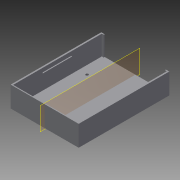
# Autodesk Inventor part: bottom1
Saved by Autodesk Inventor 2015 SP2 (Build 190223200, 223)
## iProperties
Created: 2016-03-10
Part Number: bottom1
Material: Generic
Document SubType Name: Modeling
Designer: mca20
Density: 1 g/cm^3
Appearance: Default
Author: mca20
Autodesk Inventor part; units mm, degrees
ref_plane "YZ Plane" through (0, 0, 0) normal (1, 0, 0) x (0, 1, 0)
ref_plane "XZ Plane" through (0, 0, 0) normal (0, 1, 0) x (-1, 0, 0)
ref_plane "XY Plane" through (0, 0, 0) normal (0, 0, 1) x (1, 0, 0)
sketch "Sketch1" plane through (0, 0, 0) normal (0, 1, 0) x (-1, 0, 0)
  line L0 (0, 0) -> (56, 0)
  line L1 (56, 0) -> (56, -85)
  line L2 (56, -85) -> (0, -85)
  line L3 (0, -85) -> (0, 0)
  line L4 (61, -90) -> (61, 5)
  line L5 (61, 5) -> (-5, 5)
  line L6 (-5, 5) -> (-5, -90)
  line L7 (61, -85) -> (-5, -85)
  dimension "d0" = 56
  dimension "d1" = 85
  dimension "d2" = 5
  dimension "d50" = 90
  constraints: 16 end point, 3 parallel, 3 point on line, 2 perpendicular, 1 horizontal, 2 other
  measures "d0" distance of L1.end L2.end
  measures "d1" distance of L0.end L1.end
  measures "d2" distance between parallel lines of L1 L4
  measures "d50" distance between parallel lines of L5 L2
extrude "Extrusion1" add sketch "Sketch1" along normal blind 1
sketch "Sketch2" plane through (0, 1, 0) normal (0, 1, 0) x (1, 0, 0)
  line L0 (-61, -5) -> (5, -5) projected
  line L1 (-61, 85) -> (-61, -5) projected
  line L2 (-61, -5) -> (5, -5) projected
  line L3 (5, -5) -> (5, 85) projected
  line L4 (5, 85) -> (-61, 85) projected
  line L5 (-62, 86) -> (6, 86)
  line L6 (6, 86) -> (6, -6)
  line L7 (6, -6) -> (-62, -6)
  line L8 (-62, -6) -> (-62, 86)
  point P0 (0, 0)
  dimension "d41" = 1
  constraints: 8 end point, 3 other
  measures "d41" distance between parallel lines of L4 L5
sketch "Sketch4" plane through (0, 1, 0) normal (0, 1, 0) x (1, 0, 0)
  line L0 (0, 0) -> (-56, 0)
  line L1 (-56, 0) -> (-56, 85)
  line L2 (-56, 85) -> (0, 85)
  line L3 (0, 85) -> (0, 0)
  circle A0 centre (-3.5, 3.5) radius 1.375
  circle A1 centre (-52.5, 3.5) radius 1.375
  circle A2 centre (-52.5, 61.5) radius 1.375
  circle A3 centre (-3.5, 61.5) radius 1.375
  circle A4 centre (-52.5, 3.5) radius 3.1
  circle A5 centre (-52.5, 61.5) radius 3.1
  circle A6 centre (-3.5, 3.5) radius 3.1
  circle A7 centre (-3.5, 61.5) radius 3.1
  dimension "d14" = 56
  dimension "d15" = 85
  dimension "d16" = 2.75
  dimension "d17" = 2.75
  dimension "d18" = 2.75
  dimension "d19" = 2.75
  dimension "d20" = 49
  dimension "d21" = 58
  dimension "d22" = 58
  dimension "d23" = 49
  dimension "d24" = 6.2
  dimension "d25" = 6.2
  dimension "d26" = 6.2
  dimension "d27" = 6.2
  dimension "d28" = 3.5
  dimension "d29" = 3.5
  dimension "d30" = 3.5
  dimension "d31" = 3.5
  dimension "d32" = 3.5
  constraints: 8 centre point, 8 end point, 4 coincident, 2 parallel, 1 horizontal, 1 perpendicular
  measures "d14" distance of L1.end L2.end
  measures "d15" distance of L0.end L1.end
  measures "d16" diameter of A0
  measures "d17" diameter of A1
  measures "d18" diameter of A2
  measures "d19" diameter of A3
  measures "d20" distance of A0.centre A1.centre
  measures "d21" distance of A2.centre A1.centre
  measures "d22" distance of A3.centre A0.centre
  measures "d23" distance of A3.centre A2.centre
  measures "d24" diameter of A4
  measures "d25" diameter of A5
  measures "d26" diameter of A6
  measures "d27" diameter of A7
  measures "d28" distance from line of A4.centre L1
  measures "d29" distance from line of L0 A0.centre
  measures "d30" distance from line of A2.centre L1
  measures "d31" distance from line of L3 A3.centre
  measures "d32" distance from line of L0 A1.centre
hole "Hole1" at (-52.5, 1, -61.5) at (-52.5, 1, -3.5) at (-3.5, 1, -3.5) at (-3.5, 1, -61.5) direction (0, -1, 0) diameter 2.75 end through all
extrude "Extrusion4" add sketch "Sketch2" along normal blind 20 and the other way blind 1
sketch "Sketch5" plane through (6, 21, -86) normal (0, 0, -1) x (-1, 0, 0)
  line L0 (67, -20) -> (1, -20) projected
  line L1 (68, 0) -> (0, 0) projected
  line L2 (3, -20) -> (65, -20)
  line L3 (65, -20) -> (65, 0)
  line L4 (65, 0) -> (3, 0)
  line L5 (3, 0) -> (3, -20)
  line L6 (67, 0) -> (67, -20) projected
  line L7 (1, 0) -> (1, -20) projected
  point P0 (6, -21)
  dimension "d46" = 2
  dimension "d47" = 2
  constraints: 8 end point, 2 parallel, 2 point on line, 1 horizontal, 1 perpendicular
  measures "d46" distance between parallel lines of L3 L6
  measures "d47" distance between parallel lines of L7 L5
extrude "Extrusion5" cut sketch "Sketch5" against normal blind 2 contours L0 L5 L1 L3
sketch "Sketch6" plane through (6, 0, -86) normal (1, 0, 0) x (0, 0, -1)
  line L0 (0, 21) -> (0, 0) projected
  line L1 (-92, 21) -> (0, 21) projected
  line L2 (-92, 21) -> (-92, 0) projected
  line L3 (0, 0) -> (-92, 0) projected
  point P0 (-86, 0)
extrude "Extrusion6" add sketch "Sketch6" along normal blind 0.5
sketch "Sketch7" plane through (-62, 0, 6) normal (-1, 0, 0) x (0, 0, 1)
  line L0 (0, 21) -> (0, 0) projected
  line L1 (-92, 21) -> (0, 21) projected
  line L2 (-92, 0) -> (-92, 21) projected
  line L3 (0, 0) -> (-92, 0) projected
  point P0 (-6, 0)
extrude "Extrusion7" add sketch "Sketch7" along normal blind 0.5
sketch "Sketch8" plane through (0, 21, 0) normal (0, 1, 0) x (1, 0, 0)
  line L0 (6.5, -6) -> (-62.5, -6) projected
  line L1 (6.5, 86) -> (6.5, -6) projected
  line L2 (-62.5, -6) -> (-62.5, 86) projected
  line L3 (-59, 86) -> (3, 86) projected
  line L4 (-59, 86) -> (-62.5, 86) projected
  line L5 (3, 86) -> (6.5, 86) projected
  point P0 (0, 0)
  dimension "d55" = 92
  dimension "d56" = 69
  measures "d55" distance between parallel lines of L0 L4
  measures "d56" distance between parallel lines of L1 L2
sketch "Sketch9" plane through (-61, 1, 5) normal (1, 0, 0) x (0, 0, -1)
  line L0 (0, 0) -> (0, 20) projected
  line L1 (90, 20) -> (90, 0) projected
  line L2 (0, 20) -> (90, 20) projected
  line L3 (30, 16) -> (60, 16)
  line L4 (60, 16) -> (60, 15)
  line L5 (60, 15) -> (30, 15)
  line L6 (30, 15) -> (30, 16)
  point P0 (5, -1)
  point P1 (0, 16)
  point P2 (90, 15)
  dimension "d62" = 4
  dimension "d63" = 1
  dimension "d64" = 30
  dimension "d65" = 30
  dimension "d66" = 30
  constraints: 8 end point, 2 parallel, 2 point on line, 1 horizontal, 1 perpendicular
  measures "d62" distance between parallel lines of L3 L2
  measures "d63" distance between parallel lines of L5 L3
  measures "d64" distance between parallel lines of L0 L6
  measures "d65" distance between parallel lines of L4 L1
  measures "d66" distance between parallel lines of L4 L6
extrude "Extrusion8" cut sketch "Sketch9" against normal blind 1
ref_plane "Work Plane2" through (-28, 0, -86) normal (1, 0, 0) x (0, 0, -1)
mirror "Mirror1" about plane through (-28, 0, -86) normal (1, 0, 0) of "Extrusion8"
equation "\"d22\" = d21"
equation "\"d23\" = d20"
body "Solid1"
